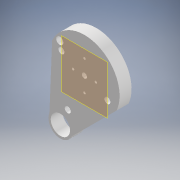
# Autodesk Inventor part: DriblerWall
Saved by Autodesk Inventor 2020 (Build 240168000, 168)
## iProperties
Created: 2025-01-13
Part Number: DriblerWall
Material: Типовые
Document SubType Name: Modeling
Designer: Ivan
Density: 1 g/cm^3
Appearance: Темно-красный
Author: Ivan
Autodesk Inventor part; units mm, degrees
ref_plane "YZ Plane" through (0, 0, 0) normal (1, 0, 0) x (0, 1, 0)
ref_plane "XZ Plane" through (0, 0, 0) normal (0, 1, 0) x (-1, 0, 0)
ref_plane "XY Plane" through (0, 0, 0) normal (0, 0, 1) x (1, 0, 0)
ref_plane "РабПлоскость1" through (0, 0, 0) normal (0, 0, 1) x (1, 0, 0)
sketch "Эскиз1" plane through (0, 0, 0) normal (0, 0, 1) x (1, 0, 0)
  circle A0 centre (0, 0) radius 15 projected
  circle A1 centre (-9.5, 0) radius 1.0064 projected
  circle A2 centre (0, -12.5) radius 1.0064 projected
  circle A3 centre (0, 12.5) radius 1.0064 projected
  circle A4 centre (9.5, 0) radius 1.0064 projected
  circle A5 centre (0, 0) radius 2 projected
  circle A6 centre (0, 0) radius 2.15
  circle A7 centre (-16.5815, 12.0542) radius 3
  circle A8 centre (-10.1413, -32.4523) radius 8.075
  circle A9 centre (-19.85, 6.2031) radius 2.5
  circle A10 centre (-5, -16) radius 2.5
  circle A11 centre (19.85, -6.2031) radius 2.5
  line L0 (19.85, -6.2031) -> (-19.85, 6.2031) construction
  line L1 (-10.1413, -32.4523) -> (-5, -16) construction
  circle A12 centre (-10.1413, -32.4523) radius 4 construction
  circle A13 centre (-10.1413, -32.4523) radius 12.5 construction
  circle A14 centre (-10.1413, -32.4523) radius 10
  line L2 (-0.5965, -35.4351) -> (-19.6861, -29.4696) construction
  circle A15 centre (0, 0) radius 24.5
  circle A16 centre (-16.5815, 12.0542) radius 4 construction
  line L3 (-0.5965, -35.4351) -> (23.3848, -7.3077)
  line L4 (-19.6861, -29.4696) -> (-23.3848, 7.3077)
  point P0 (-19.6861, -29.4696)
  dimension "d9" = 20
  dimension "d0" = 4.3
  dimension "d1" = 6
  dimension "d2" = 16.15
  dimension "d3" = 5
  dimension "d4" = 5
  dimension "d5" = 5
  dimension "d6" = 8
  dimension "d7" = 25
  dimension "d8" = 34
  dimension "d10" = 8
  dimension "d11" = 49
  constraints: 10 centre point, 10 end point, 8 coincident, 3 point on line, 2 midpoint, 2 point on circle, 1 parallel, 1 perpendicular, 1 tangent, 3 other
  measures "d0" diameter of A6
  measures "d1" diameter of A7
  measures "d2" diameter of A8
  measures "d3" diameter of A9
  measures "d4" diameter of A10
  measures "d5" diameter of A11
  measures "d6" diameter of A12
  measures "d7" diameter of A13
  measures "d8" distance from line of L1.start L0
  measures "d10" diameter of A16
  measures "d11" diameter of A15
extrude "Выдавливание1" add sketch "Эскиз1" against normal blind 11.5 contours A0 A10 | A14 A15 | L4 A15 A14 | A14 A15 L3 | A15 L4 L3 A14 | A14 A15 picked at (3.8404, -8.3906)
